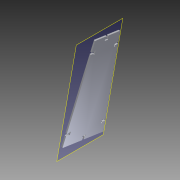
# Autodesk Inventor part: Panel_side
Saved by Autodesk Inventor 2013 (Build 170138000, 138)
## iProperties
Created: 2013-02-02
Part Number: Panel_side
Material: Aluminum 6061
Document SubType Name: Modeling
Designer: xylzlyx
Density: 1 g/cm^3
Author: xylzlyx
Autodesk Inventor part; units mm, degrees
ref_plane "YZ Plane" through (0, 0, 0) normal (1, 0, 0) x (0, 1, 0)
ref_plane "XZ Plane" through (0, 0, 0) normal (0, 1, 0) x (-1, 0, 0)
ref_plane "XY Plane" through (0, 0, 0) normal (0, 0, 1) x (1, 0, 0)
ref_plane "Work Plane1" through (-221.4413, -90.9255, -118.1004) normal (-0.9848078, 0.1736482, 0) x (-0.1736482, -0.9848078, 0)
sketch "Sketch1" plane through (-221.4413, -90.9255, -118.1004) normal (-0.9848078, 0.1736482, 0) x (-0.1736482, -0.9848078, 0)
  line L0 (0, 0) -> (-0.5513, 3.1268) construction
  line L1 (-0.5513, 3.1268) -> (245.7896, 46.5633) construction
  line L2 (245.7896, 46.5633) -> (246.341, 43.4366) construction
  line L3 (246.341, 43.4366) -> (0, 0) construction
  line L4 (254.4978, -57.6752) -> (251.371, -58.2265) construction
  line L5 (251.371, -58.2265) -> (233.8339, 41.2312) construction
  line L6 (233.8339, 41.2312) -> (236.9607, 41.7826) construction
  line L7 (236.9607, 41.7826) -> (254.4978, -57.6752) construction
  line L8 (12.5071, 2.2053) -> (23.1628, -58.2265) construction
  line L9 (23.1628, -58.2265) -> (20.0361, -58.7779) construction
  line L10 (20.0361, -58.7779) -> (9.3803, 1.654) construction
  line L11 (9.3803, 1.654) -> (12.5071, 2.2053) construction
  line L12 (264.2669, -61.4015) -> (10.2669, -61.4015) construction
  line L13 (10.2669, -61.4015) -> (10.2669, -58.2265) construction
  line L14 (10.2669, -58.2265) -> (264.2669, -58.2265) construction
  line L15 (264.2669, -58.2265) -> (264.2669, -61.4015) construction
  line L16 (233.8339, 41.2312) -> (251.371, -58.2265)
  line L17 (251.371, -58.2265) -> (23.1628, -58.2265)
  line L18 (23.1628, -58.2265) -> (12.5071, 2.2053)
  line L19 (12.5071, 2.2053) -> (233.8339, 41.2312)
  point P0 (-127.997, 118.1004)
  constraints: 40 end point, 4 collinear, 2 horizontal, 2 vertical, 28 other
extrude "SidePanel" add sketch "Sketch1" against normal blind 3.175
fillet "CornerFillet" radius 1 4 edges at (-263.5281, -338.7532, -176.327) (-260.4828, -321.4826, -76.8692) (-223.9001, -114.0121, -176.327) (-222.0498, -103.5182, -115.8951)
sketch "ScrewSketch" plane through (-221.4413, -90.9255, -118.1004) normal (-0.9848078, 0.1736482, 0) x (0, 0, 1)
  line L0 (1.2205, -12.6807) -> (-57.4002, -23.0171) projected
  line L1 (-57.0529, -251.164) -> (40.2464, -234.0076) projected
  line L2 (41.0576, -232.8491) -> (2.379, -13.4919) projected
  line L3 (-61.4015, -11.2669) -> (-61.4015, -263.2669) projected
  line L4 (-58.2265, -250.1792) -> (-58.2265, -24.0019) projected
  line L5 (-61.4015, -225.764) -> (-48.7015, -225.764)
  line L6 (-61.4015, -221.9667) -> (-48.7015, -221.9667)
  line L7 (-61.4015, -221.9667) -> (-61.4015, -225.764)
  line L8 (-48.7015, -225.764) -> (-48.7015, -221.9667)
  line L9 (-61.4015, -48.4171) -> (-48.7015, -48.4171)
  line L10 (-48.7015, -48.4171) -> (-48.7015, -52.2144)
  line L11 (-48.7015, -52.2144) -> (-61.4015, -52.2144)
  line L12 (-61.4015, -52.2144) -> (-61.4015, -48.4171)
  line L13 (3.3004, -0.4335) -> (46.3897, -244.8048) projected
  line L14 (-2.7643, -39.1752) -> (9.7428, -36.9698)
  line L15 (-2.7643, -39.1752) -> (-2.1049, -42.9148)
  line L16 (-2.1049, -42.9148) -> (10.4022, -40.7095)
  line L17 (10.4022, -40.7095) -> (9.7428, -36.9698)
  line L18 (27.4403, -210.4738) -> (39.9473, -208.2685)
  line L19 (27.4403, -210.4738) -> (26.7809, -206.7342)
  line L20 (26.7809, -206.7342) -> (39.2879, -204.5288)
  line L21 (39.2879, -204.5288) -> (39.9473, -208.2685)
  line L22 (40.7978, -237.1343) -> (-56.6904, -254.3241) projected
  line L23 (0.6692, -9.5539) -> (-57.2417, -19.7652) projected
  line L24 (-48.7015, -227.9611) -> (-48.7015, -219.7696)
  line L25 (-48.7015, -219.7696) -> (-51.7337, -219.7696)
  line L26 (-48.7015, -227.9611) -> (-51.7337, -227.9611)
  line L27 (-51.7337, -227.9611) -> (-51.7337, -219.7696)
  line L28 (-48.7015, -46.22) -> (-48.7015, -54.4115)
  line L29 (-48.7015, -54.4115) -> (-51.7337, -54.4115)
  line L30 (-51.7337, -54.4115) -> (-51.7337, -46.22)
  line L31 (-51.7337, -46.22) -> (-48.7015, -46.22)
  line L32 (-1.7234, -45.0785) -> (-3.1458, -37.0115)
  line L33 (-1.7234, -45.0785) -> (1.2627, -44.552)
  line L34 (1.2627, -44.552) -> (-0.1598, -36.4849)
  line L35 (-0.1598, -36.4849) -> (-3.1458, -37.0115)
  line L36 (27.8218, -212.6375) -> (26.3994, -204.5705)
  line L37 (26.3994, -204.5705) -> (29.3854, -204.0439)
  line L38 (29.3854, -204.0439) -> (30.8079, -212.111)
  line L39 (30.8079, -212.111) -> (27.8218, -212.6375)
  line L40 (-6.0765, -245.3995) -> (-8.2819, -232.8925)
  line L41 (-12.0215, -233.5519) -> (-9.8161, -246.0589)
  line L42 (-8.2819, -232.8925) -> (-12.0215, -233.5519)
  line L43 (-6.0765, -245.3995) -> (-9.8161, -246.0589)
  line L44 (-14.1852, -233.9334) -> (-6.1181, -232.5109)
  line L45 (-13.6587, -236.9194) -> (-14.1852, -233.9334)
  line L46 (-13.6587, -236.9194) -> (-5.5916, -235.497)
  line L47 (-5.5916, -235.497) -> (-6.1181, -232.5109)
  line L48 (-26.4165, -14.3299) -> (-24.2111, -26.8369)
  line L49 (-24.2111, -26.8369) -> (-27.9507, -27.4963)
  line L50 (-27.9507, -27.4963) -> (-30.1561, -14.9893)
  line L51 (-30.1561, -14.9893) -> (-26.4165, -14.3299)
  line L52 (-30.1145, -27.8778) -> (-22.0474, -26.4554)
  line L53 (-22.0474, -26.4554) -> (-22.5739, -23.4694)
  line L54 (-22.5739, -23.4694) -> (-30.641, -24.8918)
  line L55 (-30.641, -24.8918) -> (-30.1145, -27.8778)
  point P0 (-48.7015, -50.3158)
  point P1 (-48.7015, -223.8654)
  point P2 (-2.4346, -41.045)
  point P3 (27.1106, -208.604)
  point P4 (-7.9463, -245.7292)
  point P5 (-10.1517, -233.2222)
  point P6 (-28.2863, -14.6596)
  point P7 (-26.0809, -27.1666)
  dimension "d6" = 25.4
  dimension "d7" = 12.7
  dimension "d8" = 3.7973
  dimension "d9" = 25.4
  dimension "d10" = 12.7
  dimension "d11" = 3.7973
  dimension "d14" = 12.7
  dimension "d15" = 25.4
  dimension "d17" = 3.7973
  dimension "d18" = 12.7
  dimension "d19" = 25.4
  dimension "d20" = 3.7973
  dimension "d21" = 8.1915
  dimension "d22" = 3.0321
  dimension "d23" = 8.1915
  dimension "d24" = 3.0321
  dimension "d25" = 8.1915
  dimension "d26" = 3.0321
  dimension "d27" = 8.1915
  dimension "d28" = 3.0321
  dimension "d29" = 12.7
  dimension "d30" = 3.7973
  dimension "d31" = 8.1915
  dimension "d32" = 3.0321
  dimension "d33" = 3.7973
  dimension "d34" = 12.7
  dimension "d35" = 8.1915
  dimension "d36" = 3.0321
  constraints: 96 end point, 35 parallel, 16 midpoint, 9 collinear, 6 perpendicular, 6 point on line
  measures "d6" distance from line of L1.start L5
  measures "d7" distance of L5.start L5.end
  measures "d8" distance between parallel lines of L5 L6
  measures "d9" vertical distance of L0.end L9.start
  measures "d10" distance of L9.start L9.end
  measures "d11" distance of L11.end L9.start
  measures "d14" distance of L14.start L14.end
  measures "d15" distance between parallel lines of L0 L14
  measures "d17" distance between parallel lines of L14 L16
  measures "d18" distance of L18.start L18.end
  measures "d19" distance between parallel lines of L1 L18
  measures "d20" distance of L20.end L18.end
  measures "d21" distance of L24.start L24.end
  measures "d22" distance of L24.end L25.end
  measures "d23" distance of L28.start L28.end
  measures "d24" distance of L28.end L29.end
  measures "d25" distance of L32.start L32.end
  measures "d26" distance of L32.start L33.end
  measures "d27" distance of L36.start L36.end
  measures "d28" distance of L36.end L37.end
  measures "d29" distance of L40.start L40.end
  measures "d30" distance of L40.end L41.start
  measures "d31" distance of L44.start L44.end
  measures "d32" distance of L45.start L44.start
  measures "d33" distance of L50.end L48.start
  measures "d34" distance of L49.end L50.end
  measures "d35" distance of L52.start L52.end
  measures "d36" distance of L52.end L53.end
extrude "ScrewSlots" cut sketch "ScrewSketch" against normal blind 25.4 contours L48 L54 L50 L0 | L0 L50 L23 L48 | L54 L53 L52 L48 | L48 L49 L50 L54 | L50 L52 L55 L54 | L41 L46 L40 L1 | L1 L40 L22 L41 | L46 L45 L44 L41 | L41 L42 L40 L46 | L40 L44 L47 L46 | L18 L38 L20 L2 | L2 L20 L13 L18 | L38 L39 L36 L18 | L18 L19 L20 L38 | L16 L34 L14 L2 | L2 L14 L13 L16 | L20 L36 L37 L38 | L34 L33 L32 L16 | L16 L15 L14 L34 | L14 L32 L35 L34 | L9 L4 L11 L3 | L9 L30 L11 L4 | L6 L4 L5 L3 | L30 L31 L28 L9 | L9 L10 L11 L30 | L6 L27 L5 L4 | L11 L28 L29 L30 | L27 L25 L24 L6 | L6 L8 L5 L27 | L5 L24 L26 L27
fillet "SlotFillets" radius 0.5 48 edges at (-261.9482, -329.7932, -124.7283) (-260.8378, -323.4961, -125.8558) (-262.0627, -330.4426, -128.4679) (-260.9523, -324.1455, -129.5954) (-261.0186, -324.5212, -131.7591) (-260.5001, -321.5805, -132.2856) (-260.2531, -320.1797, -124.2186) (-260.7716, -323.1204, -123.6921) (-256.3349, -297.9588, -87.6741) (-256.7106, -300.0897, -87.2926) (-256.8021, -300.6082, -90.2787) (-255.4012, -292.6637, -91.7011) (-255.3098, -292.1452, -88.715) (-255.6855, -294.276, -88.3335) (-256.1391, -296.8485, -81.2799) (-255.4898, -293.1657, -81.9393) (-259.463, -315.699, -166.802) (-259.463, -315.699, -169.8341) (-259.0815, -313.5353, -169.8341) (-259.0815, -313.5353, -176.327) (-258.4221, -309.7957, -176.327) (-258.4221, -309.7957, -169.8341) (-258.0406, -307.632, -169.8341) (-258.0406, -307.632, -166.802) (-229.3264, -144.786, -166.802) (-229.3264, -144.786, -169.8341) (-228.9449, -142.6223, -169.8341) (-228.9449, -142.6223, -176.327) (-228.2855, -138.8827, -176.327) (-228.2855, -138.8827, -169.8341) (-227.904, -136.719, -169.8341) (-227.904, -136.719, -166.802) (-224.7189, -118.6554, -148.2149) (-224.4719, -117.2546, -140.1479) (-223.9534, -114.3139, -140.6744) (-224.0196, -114.6897, -142.8381) (-224.1341, -115.339, -146.5777) (-224.2004, -115.7148, -148.7414) (-223.0238, -109.0419, -147.7052) (-222.9093, -108.3926, -143.9656) (-226.3049, -127.6503, -121.2463) (-227.6143, -135.0763, -116.8378) (-227.7058, -135.5948, -119.8238) (-226.2135, -127.1318, -118.2602) (-226.3934, -128.1523, -111.4844) (-227.0428, -131.8351, -110.8251) (-226.5892, -129.2626, -117.8787) (-227.2386, -132.9454, -117.2193)
equation "\"d7\" = ScrewLen"
equation "\"d8\" = ScrewHoleD"
equation "\"d10\" = ScrewLen"
equation "\"d11\" = ScrewHoleD"
equation "\"d14\" = ScrewLen"
equation "\"d17\" = ScrewHoleD"
equation "\"d18\" = ScrewLen"
equation "\"d20\" = ScrewHoleD"
equation "\"d21\" = NutFlatsGap"
equation "\"d22\" = NutHeightGap"
equation "\"d23\" = NutFlatsGap"
equation "\"d24\" = NutHeightGap"
equation "\"d25\" = NutFlatsGap"
equation "\"d26\" = NutHeightGap"
equation "\"d27\" = NutFlatsGap"
equation "\"d28\" = NutHeightGap"
equation "\"d29\" = ScrewLen"
equation "\"d30\" = ScrewHoleD"
equation "\"d31\" = NutFlatsGap"
equation "\"d32\" = NutHeightGap"
equation "\"d33\" = ScrewHoleD"
equation "\"d34\" = ScrewLen"
equation "\"d35\" = NutFlatsGap"
equation "\"d36\" = NutHeightGap"
equation "\"ScrewLen\" = 12.7"
equation "\"ScrewHoleD\" = 3.7973"
equation "\"NutFlatsGap\" = 8.1915"
equation "\"NutHeightGap\" = 3.03212"
equation "\"SlotFilletRad\" = 0.5"
body "Solid1"
